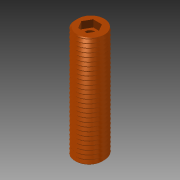
# Autodesk Inventor part: hub screw
Saved by Autodesk Inventor 2014 (Build 180170000, 170)
## iProperties
Created: 2013-10-15
Part Number: hub screw
Material: Generic
Document SubType Name: Modeling
Designer: employee
Density: 1 g/cm^3
Mass: 6.707 g
Surface Area: 44.4402 cm^2
Volume: 6.707 cm^3
Appearance: Smooth - Light Orange
Author: employee
Autodesk Inventor part; units mm, degrees
ref_plane "YZ Plane" through (0, 0, 0) normal (1, 0, 0) x (0, 1, 0)
ref_plane "XZ Plane" through (0, 0, 0) normal (0, 1, 0) x (-1, 0, 0)
ref_plane "XY Plane" through (0, 0, 0) normal (0, 0, 1) x (1, 0, 0)
sketch "Sketch1" plane through (0, 0, 0) normal (0, 0, 1) x (1, 0, 0)
  circle A0 centre (0, 0) radius 7.25
  circle A1 centre (0, 0) radius 2.5
  dimension "d0" = 14.5
  dimension "d2" = 5
  constraints: 2 centre point, 2 coincident
  measures "d0" diameter of A0
  measures "d2" diameter of A1
extrude "Extrusion1" add sketch "Sketch1" along normal blind 55
sketch "Sketch2" plane through (0, 0, 0) normal (0, 1, 0) x (-1, 0, 0)
  line L0 (7.25, 55) -> (7.25, 0) projected
  line L1 (7.25, 0) -> (2.5, 0) projected
  line L2 (2.5, 0) -> (2.5, 55) projected
  line L3 (2.5, 55) -> (7.25, 55) projected
  line L4 (-7.25, 0) -> (-7.25, 55) projected
  line L5 (-7.25, 55) -> (-2.5, 55) projected
  line L6 (-2.5, 55) -> (-2.5, 0) projected
  line L7 (-2.5, 0) -> (-7.25, 0) projected
  line L8 (-7.25, 55) -> (-7.25, 57)
  line L9 (-7.25, 57) -> (-6.25, 56)
  line L10 (-6.25, 56) -> (-7.25, 55)
  line L11 (0, 0) -> (0, 81.5152)
  dimension "d5" = 2
  constraints: 8 end point, 3 perpendicular, 1 parallel
  measures "d5" distance of L4.end L8.end
coil "Coil1" sketch "Sketch2" operation cut axis through (0, 0, 0) along (0, 0, -1) pitch 2.001 turns 30 hand right contours L8 L9 L10
sketch "Sketch3" plane through (0, 0, 55) normal (0, 0, 1) x (1, 0, 0)
  circle A0 centre (0, 0) radius 2.5 projected
  line L0 (-2.1651, 3.75) -> (2.1651, 3.75)
  line L1 (2.1651, 3.75) -> (4.3301, 0)
  line L2 (4.3301, 0) -> (2.1651, -3.75)
  line L3 (2.1651, -3.75) -> (-2.1651, -3.75)
  line L4 (-2.1651, -3.75) -> (-4.3301, 0)
  line L5 (-4.3301, 0) -> (-2.1651, 3.75)
  dimension "d14" = 7.5
  constraints: 12 end point, 1 coincident, 1 horizontal, 13 other
  measures "d14" distance between parallel lines of L3 L0
extrude "Extrusion2" cut sketch "Sketch3" against normal blind 3.5
body "Solid1"
